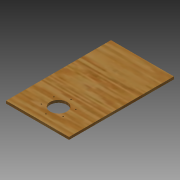
# Autodesk Inventor part: base_plate
Saved by Autodesk Inventor 2013 (Build 170138000, 138)
## iProperties
Created: 2014-10-12
Part Number: base_plate
Material: Plywood, Finish
Document SubType Name: Modeling
Designer: Masta
Density: 1 g/cm^3
Author: Masta
Autodesk Inventor part; units mm, degrees
ref_plane "YZ Plane" through (0, 0, 0) normal (1, 0, 0) x (0, 1, 0)
ref_plane "XZ Plane" through (0, 0, 0) normal (0, 1, 0) x (-1, 0, 0)
ref_plane "XY Plane" through (0, 0, 0) normal (0, 0, 1) x (1, 0, 0)
sketch "Sketch1" plane through (0, 0, 0) normal (0, 0, 1) x (1, 0, 0)
  line L0 (-75, -50) -> (75, -50)
  line L1 (75, -50) -> (75, 200)
  line L2 (75, 200) -> (-75, 200)
  line L3 (-75, 200) -> (-75, -50)
  circle A0 centre (0, 0) radius 20
  line L4 (0, 0) -> (0, 30) construction
  dimension "d0" = 150
  dimension "d1" = 250
  dimension "d2" = 40
  dimension "d16" = 30
  dimension "d17" = 50
  constraints: 10 end point, 3 parallel, 2 coincident, 1 centre point, 1 horizontal, 1 perpendicular, 1 other
  measures "d0" distance of L2.end L1.end
  measures "d1" distance of L1.end L0.end
  measures "d2" diameter of A0
  measures "d16" distance of L4.start L4.end
  measures "d17" distance from line of L0 point (0, 0)
extrude "Extrusion1" add sketch "Sketch1" along normal blind 6
hole "Hole1" at (0, 30, 0) direction (0, 0, 1) diameter 3 end through all
pattern_circular "Circular Pattern1" count 6 over 360 about axis through (0, 0, 0) along (0, 0, 1) of "Hole1"
body "Solid1"
